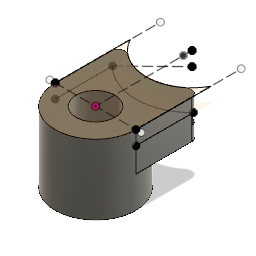
Piezo_mount_on_small_solenoid (Autodesk Fusion 360 design; units mm, degrees)
Autodesk Fusion 360 part; units mm, degrees
sketch "Sketch1" plane through (0, 0, 0) normal (0, 1, 0) x (1, 0, 0)
  circle A0 centre (0, 0) radius 2.75
  circle A1 centre (0, 0) radius 5.75
  line L0 (-6, 0) -> (6, 0) construction
  dimension "d1" = 5.5
  dimension "d2" = 3
  measures "d1" diameter of A0
extrude "Extrude1" add sketch "Sketch1" against normal blind 10
sketch "Sketch2" plane through (0, 0, 0) normal (0, 1, 0) x (-1, 0, 0)
  circle A0 centre (0, 0) radius 2.75
  circle A1 centre (0, 0) radius 5.75
  line L0 (-6.5, 0) -> (6.5, 0) construction
  line L1 (0, -13.75) -> (0, 0) construction
  line L2 (-5.75, 0) -> (-5.75, -15) construction
  line L3 (5.75, 0) -> (5.75, -15) construction
  arc A2 (5.75, -10.7189) -> (0, -7.25) centre (0, -13.75) ccw
  arc A3 (0, -7.25) -> (-5.75, -10.7189) centre (0, -13.75) ccw
  line L4 (-5.75, -10.7189) -> (-5.75, 0)
  line L5 (5.75, -10.7189) -> (5.75, 0)
  dimension "d16" = 13.75
  dimension "d17" = 6.5
  measures "d16" distance of A0.centre
  measures "d17" radius of A2
extrude "Extrude3" add sketch "Sketch2" against normal blind 2 contours A1 A2 A3 L4 L5
sketch "Sketch3" plane through (0, -2, 0) normal (0, -1, 0) x (1, 0, 0)
  arc A0 (5.75, -10.7189) -> (-5.75, -10.7189) centre (0, -13.75) ccw
  line L0 (5.75, -10.7189) -> (5.75, 0)
  arc A1 (-5.75, 0) -> (5.75, 0) centre (0, 0) ccw
  line L1 (-5.75, 0) -> (-5.75, -10.7189)
  arc A2 (5.75, -8.1879) -> (0, -5.75) centre (0, -13.75) ccw
  arc A3 (0, -5.75) -> (-5.75, -8.1879) centre (0, -13.75) ccw
  line L2 (-5.75, 0) -> (-5.75, -8.1879)
  line L3 (5.75, 0) -> (5.75, -8.1879)
  line L4 (-5.75, -8.1879) -> (0, -13.75) construction
  dimension "d24" = 8
extrude "Extrude4" add sketch "Sketch3" along normal blind 1.5 contours L0 A1 A2 L3 | A1 L1 A3 L2
sketch "Sketch5" plane through (0, -3.5, 0) normal (0, -1, 0) x (1, 0, 0)
  arc A0 (-5.75, 0) -> (0, -5.75) centre (0, 0) ccw
  line L0 (-5.75, 0) -> (-5.75, -8.1879)
  arc A1 (0, -5.75) -> (-5.75, -8.1879) centre (0, -13.75) ccw
  arc A2 (0, -7.25) -> (-5.75, -10.7189) centre (0, -13.75) ccw
  arc A3 (5.75, -10.7189) -> (0, -7.25) centre (0, -13.75) ccw
  line L1 (-5.75, -10.7189) -> (-5.75, 0)
  circle A4 centre (0, 0) radius 5.75
  line L2 (5.75, -10.7189) -> (5.75, 0)
  line L3 (0, -13.75) -> (0, 0)
  line L4 (0, -13.75) -> (-2.9897, -7.9784) construction
  dimension "d25" = 6.5
extrude "Extrude5" add sketch "Sketch5" along normal blind 2 contours A0 L0 A1 L1 A4 | A1 A2 L1 L3 | A3 A4 L2 L3
fillet "Fillet2" radius 1 2 edges at (5.75, -1, -10.7189) (5.75, -4.5, -10.7189)
fillet "Fillet4" radius 1 2 edges at (-5.75, -1, -10.7189) (-5.75, -4.5, -10.7189)
